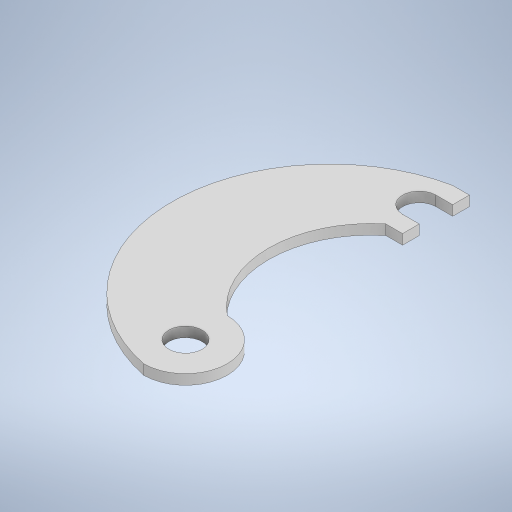
# Autodesk Inventor part: key
Saved by Autodesk Inventor 2023 (Build 270158030, 158C)
## iProperties
Created: 2023-03-06
Part Number: key
Material: Generic
Document SubType Name: Modeling
Designer: fatih
Density: 1 g/cm^3
Appearance: Default
Author: fatih
Autodesk Inventor part; units mm, degrees
ref_plane "YZ Plane" through (0, 0, 0) normal (1, 0, 0) x (0, 1, 0)
ref_plane "XZ Plane" through (0, 0, 0) normal (0, 1, 0) x (-1, 0, 0)
ref_plane "XY Plane" through (0, 0, 0) normal (0, 0, 1) x (1, 0, 0)
sketch "Sketch1" plane through (0, 0, 0) normal (0, 1, 0) x (-1, 0, 0)
  circle A0 centre (0, 0) radius 5
  arc A1 (0, 12.5) -> (0, -12.5) centre (0, 0) ccw
  line L0 (0, 0) -> (0, -70)
  arc A2 (0, -75) -> (0, -65) centre (0, -70) ccw
  arc A3 (0, -80) -> (4.8696, -78.7342) centre (0, -70) ccw
  arc A4 (0, -80) -> (0, 12.5) centre (-9.4226, -33.75) ccw
  arc A5 (0, -60) -> (0, -12.5) centre (-19.2794, -36.25) ccw
  line L1 (0, -60) -> (-5, -60)
  line L2 (0, -65) -> (-5, -65)
  line L3 (0, -75) -> (-5, -75)
  line L4 (0, -60) -> (0, -65)
  line L5 (0, -75) -> (0, -80)
  line L6 (-5, -60) -> (-5, -65)
  line L7 (-5, -75) -> (-5, -80)
  line L8 (0, -80) -> (0, -75)
  line L9 (0, -65) -> (0, -60)
  line L10 (0, -80) -> (-5, -80)
  dimension "d0" = 10
  dimension "d1" = 25
  dimension "d2" = 70
  dimension "d3" = 10
  dimension "d4" = 20
  dimension "d5" = 5
  constraints: 22 end point, 11 point on circle, 7 perpendicular, 6 centre point, 4 coincident, 4 parallel, 3 vertical, 2 point on line, 1 horizontal
  measures "d0" diameter of A0
  measures "d1" diameter of A1
  measures "d2" distance of L0.start L0.end
  measures "d3" diameter of A2
  measures "d4" diameter of A3
  measures "d5" distance of L5.end L7.end
extrude "Extrusion1" add sketch "Sketch1" along normal blind 3 contours A4 L5 A2 L0 A5 A1 | L0 L2 L6 L1 | L10 L7 L3 L5
body "Solid1"
